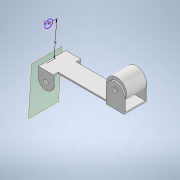
# Autodesk Inventor part: Arm
Saved by Autodesk Inventor 2020 (Build 240168000, 168)
## iProperties
Created: 2019-04-17
Part Number: Arm
Material: Generic
Document SubType Name: Modeling
Designer: Parker
Density: 1 g/cm^3
Appearance: Default
Author: Parker
Autodesk Inventor part; units mm, degrees
ref_plane "YZ Plane" through (0, 0, 0) normal (1, 0, 0) x (0, 1, 0)
ref_plane "XZ Plane" through (0, 0, 0) normal (0, 1, 0) x (-1, 0, 0)
ref_plane "XY Plane" through (0, 0, 0) normal (0, 0, 1) x (1, 0, 0)
sketch "Sketch1" plane through (0, 0, 0) normal (1, 0, 0) x (0, 1, 0)
  line L0 (1.75, 3.05) -> (-2.05, 3.05)
  line L1 (-2.05, 3.05) -> (-2.05, 2.75)
  line L2 (-2.05, 2.75) -> (1.45, 2.75)
  line L3 (1.45, 2.75) -> (1.45, -2.75)
  line L4 (1.45, -2.75) -> (-2.05, -2.75)
  line L5 (-2.05, -2.75) -> (-2.05, -3.05)
  line L6 (-2.05, -3.05) -> (1.75, -3.05)
  line L7 (1.75, -3.05) -> (1.75, 3.05)
  point P0 (0, 0)
  dimension "d0" = 0.3
  dimension "d1" = 0.3
  dimension "d2" = 0.3
  dimension "d4" = 3.5
  dimension "d15" = 6.1
  dimension "d16" = 3.05
  dimension "d17" = 1.75
  constraints: 16 end point, 6 perpendicular, 2 point on line, 1 horizontal
  measures "d0" distance of L0.end L1.end
  measures "d1" distance of L4.end L5.end
  measures "d2" distance between parallel lines of L7 L3
  measures "d4" distance of L1.end L2.end
  measures "d15" distance between parallel lines of L6 L0
  measures "d16" distance from line of point (0, 0) L6
  measures "d17" distance from line of point (0, 0) L7
extrude "Extrusion1" add sketch "Sketch1" along normal blind 3.3
fillet "Fillet1" radius 1.6 4 edges at (3.3, -2.05, 2.9) (0, -2.05, 2.9) (0, -2.05, -2.9) (3.3, -2.05, -2.9)
sketch "Sketch2" plane through (0, 1.75, 3.05) normal (0, 0, 1) x (1, 0, 0)
  arc A0 (1.7, -3.8) -> (3.3, -2.2) centre (1.7, -2.2) ccw projected
  arc A1 (0, -2.2) -> (1.6, -3.8) centre (1.6, -2.2) ccw projected
  line L0 (1.6, -2.2) -> (1.7, -2.2)
  point P0 (0, -1.75)
  point P1 (1.65, -2.2)
  constraints: 2 end point, 1 horizontal, 1 midpoint
hole "Hole1" at (1.65, -0.45, 3.05) direction (0, 0, -1) diameter 1 end through all
sketch "Sketch3" plane through (3.3, 0, 0) normal (1, 0, 0) x (0, 0, -1)
  line L0 (3.05, 1.75) -> (-3.05, 1.75) projected
  line L1 (0, 1.75) -> (0, 1.45)
  line L2 (-2.75, 1.45) -> (2.75, 1.45) projected
  line L3 (2, 1.45) -> (-2, 1.45)
  line L4 (-2, 1.45) -> (-2, 1.75)
  line L5 (-2, 1.75) -> (2, 1.75)
  line L6 (2, 1.75) -> (2, 1.45)
  line L7 (2, 1.45) -> (-2, 1.75) construction
  line L8 (-2, 1.45) -> (2, 1.75) construction
  point P0 (0, 0)
  point P1 (0, 1.6)
  dimension "d18" = 4
  constraints: 14 end point, 5 midpoint, 2 parallel, 1 horizontal, 1 perpendicular, 1 point on line
  measures "d18" distance between parallel lines of L6 L4
extrude "Extrusion2" add sketch "Sketch3" along normal blind 15.25
sketch "Sketch4" plane through (18.55, 0, 0) normal (1, 0, 0) x (0, 0, -1)
  line L0 (-2.75, 1.45) -> (2.75, 1.45) projected
  line L1 (0, 1.45) -> (0, 1.75)
  line L2 (3.05, 1.75) -> (-3.05, 1.75) projected
  line L3 (2.5, 1.45) -> (-2.5, 1.45)
  line L4 (-2.5, 1.45) -> (-2.5, 1.75)
  line L5 (-2.5, 1.75) -> (2.5, 1.75)
  line L6 (2.5, 1.75) -> (2.5, 1.45)
  line L7 (2.5, 1.45) -> (-2.5, 1.75) construction
  line L8 (-2.5, 1.45) -> (2.5, 1.75) construction
  line L9 (-2.5, 1.75) -> (-2.2, 1.75)
  line L10 (-2.2, 1.75) -> (-2.2, 6.75)
  line L11 (-2.2, 6.75) -> (-2.5, 6.75)
  line L12 (-2.5, 6.75) -> (-2.5, 1.75)
  line L13 (2.5, 1.75) -> (2.2, 1.75)
  line L14 (2.2, 1.75) -> (2.2, 6.75)
  line L15 (2.2, 6.75) -> (2.5, 6.75)
  line L16 (2.5, 6.75) -> (2.5, 1.75)
  point P0 (0, 0)
  point P1 (0, 1.6)
  dimension "d21" = 5
  dimension "d22" = 0.3
  dimension "d23" = 0.3
  dimension "d24" = 5
  constraints: 30 end point, 6 parallel, 5 midpoint, 3 horizontal, 3 perpendicular, 2 point on line
  measures "d21" distance between parallel lines of L6 L4
  measures "d22" distance of L14.end L15.end
  measures "d23" distance of L10.end L11.end
  measures "d24" distance of L9.end L10.end
extrude "Extrusion3" add sketch "Sketch4" against normal blind 4
fillet "Fillet2" radius 2 4 edges at (18.55, 6.75, 2.35) (14.55, 6.75, 2.35) (14.55, 6.75, -2.35) (18.55, 6.75, -2.35)
sketch "Sketch5" plane through (14.55, 1.45, 2.5) normal (0, 0, 1) x (1, 0, 0)
  arc A0 (4, 3.3) -> (0, 3.3) centre (2, 3.3) ccw projected
  point P0 (-14.55, -1.45)
  point P1 (2, 3.8)
  dimension "d35" = 0.5
  measures "d35" distance of A0.centre point (2, 3.8)
hole "Hole2" at (16.55, 5.25, 2.5) direction (0, 0, -1) diameter 1 end through all
sketch "Sketch6" plane through (14.55, 1.75, -2.2) normal (0, 0, 1) x (1, 0, 0)
  circle A0 centre (2, 3.5) radius 0.5 projected
  circle A1 centre (2, 3.5) radius 0.5 projected
  circle A2 centre (2, 3.5) radius 2.25
  point P0 (-14.55, -1.75)
  dimension "d36" = 4.5
  constraints: 1 centre point, 1 coincident
  measures "d36" diameter of A2
extrude "Extrusion4" add sketch "Sketch6" along normal blind 4.4 contours A0 | A2
ref_plane "Work Plane1" through (-1.2438, 1.2458, -3.05) normal (-0.9978, 0.0664, 0) x (-0.0664, -0.9978, 0)
sketch "Sketch7" plane through (-1.2438, 1.2458, -3.05) normal (-0.9978, 0.0664, 0) x (-0.0664, -0.9978, 0)
  circle A0 centre (-6.8395, 3.05) radius 0.875
  point P0 (1.1605, 3.05)
  dimension "d39" = 1.75
  dimension "d40" = 8
  constraints: 1 centre point
  measures "d39" diameter of A0
  measures "d40" distance of point (1.16, 3.05) A0.centre
body "Solid1"
